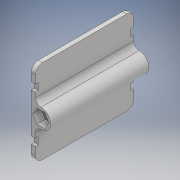
# Autodesk Inventor part: Soporte ESC
Saved by Autodesk Inventor 2019 (Build 230136000, 136)
## iProperties
Part Number: Soporte ESC
Material: Genérico
Document SubType Name: Modeling
Designer: beta3
Density: 1 g/cm^3
Appearance: Valor por defecto
Author: beta3
Autodesk Inventor part; units mm, degrees
ref_plane "YZ Plane" through (0, 0, 0) normal (1, 0, 0) x (0, 1, 0)
ref_plane "XZ Plane" through (0, 0, 0) normal (0, 1, 0) x (-1, 0, 0)
ref_plane "XY Plane" through (0, 0, 0) normal (0, 0, 1) x (1, 0, 0)
sketch "Boceto1" plane through (0, 0, 0) normal (0, 1, 0) x (-1, 0, 0)
  circle A0 centre (0, 0) radius 3.15
  line L0 (6.889, 30) -> (3.889, 30)
  line L1 (3.889, -30) -> (6.889, -30)
  line L2 (6.889, -30) -> (6.889, 30)
  line L3 (0, 0) -> (3.15, 0) construction
  arc A1 (0, 6.889) -> (0, -6.889) centre (0, 0) ccw
  line L4 (3.889, 30) -> (3.889, 10.7779)
  line L5 (3.889, -30) -> (3.889, -10.7779)
  arc A2 (0, 6.889) -> (3.889, 10.7779) centre (0, 10.7779) ccw
  arc A3 (3.889, -10.7779) -> (0, -6.889) centre (0, -10.7779) ccw
  line L6 (2.9445, 5.1) -> (5.889, 0) construction
  line L7 (5.889, 0) -> (2.9445, -5.1) construction
  line L8 (2.9445, -5.1) -> (-2.9445, -5.1) construction
  line L9 (-2.9445, -5.1) -> (-5.889, 0) construction
  line L10 (-5.889, 0) -> (-2.9445, 5.1) construction
  line L11 (-2.9445, 5.1) -> (2.9445, 5.1) construction
  line L12 (5.889, 0) -> (6.889, 0) construction
  line L13 (-5.889, 0) -> (-6.889, 0) construction
  line L14 (0, -10.7779) -> (0, 0) construction
  dimension "d0" = 6.3
  dimension "d3" = 10.2
  dimension "d4" = 1
  dimension "d5" = 3
  dimension "d12" = 60
  constraints: 30 end point, 7 point on circle, 4 symmetric about line, 4 tangent, 3 centre point, 3 coincident, 3 horizontal, 3 vertical, 1 collinear, 1 horizontal alignment, 1 midpoint, 1 parallel, 15 other
  measures "d3" distance between parallel lines of L8 L11
  measures "d4" distance of L6.end L12.end
  measures "d5" distance of L1.start L1.end
  measures "d12" distance of L1.end L0.start
extrude "Extrusión1" add sketch "Boceto1" along normal blind 70
sketch "Boceto2" plane through (0, 0, 0) normal (0, -1, 0) x (1, 0, 0)
  line L0 (-5.7735, 0) -> (-2.8868, 5)
  line L1 (-2.8868, 5) -> (2.8868, 5)
  line L2 (2.8868, 5) -> (5.7735, 0)
  line L3 (5.7735, 0) -> (2.8868, -5)
  line L4 (2.8868, -5) -> (-2.8868, -5)
  line L5 (-2.8868, -5) -> (-5.7735, 0)
  point P0 (0, 0)
  point P1 (0, 0)
  dimension "d8" = 10
  constraints: 12 end point, 1 coincident, 13 other
  measures "d8" distance between parallel lines of L4 L1
extrude "Extrusión2" cut sketch "Boceto2" against normal blind 6
sketch "Boceto4" plane through (-6.889, 0, -30) normal (-1, 0, 0) x (0, 0, 1)
  line L0 (10.7549, 2) -> (15.7549, 2)
  line L1 (15.7549, 2) -> (15.7549, 0)
  line L2 (15.7549, 0) -> (10.7549, 0)
  line L3 (10.7549, 0) -> (10.7549, 2)
  line L4 (44.2451, 2) -> (49.2451, 2)
  line L5 (49.2451, 2) -> (49.2451, 0)
  line L6 (49.2451, 0) -> (44.2451, 0)
  line L7 (44.2451, 0) -> (44.2451, 2)
  line L8 (0, 0) -> (60, 0) projected
  line L9 (30, 0) -> (30, 6) projected
  line L10 (30, 0) -> (30, 70) construction
  line L11 (0, 70) -> (60, 70) projected
  line L12 (30, 35) -> (1.5097, 35) construction
  line L13 (10.7549, 68) -> (15.7549, 68)
  line L14 (15.7549, 68) -> (15.7549, 70)
  line L15 (15.7549, 70) -> (10.7549, 70)
  line L16 (10.7549, 70) -> (10.7549, 68)
  line L17 (44.2451, 68) -> (49.2451, 68)
  line L18 (49.2451, 68) -> (49.2451, 70)
  line L19 (49.2451, 70) -> (44.2451, 70)
  line L20 (44.2451, 70) -> (44.2451, 68)
  point P0 (47.493, 22.347)
  dimension "d19" = 5
  dimension "d20" = 2
  constraints: 36 end point, 9 symmetric about line, 4 parallel, 3 horizontal, 2 equal length, 2 midpoint, 2 perpendicular, 1 point on line
  measures "d19" distance of L4.start L4.end
  measures "d20" distance of L6.end L4.start
extrude "Extrusión3" cut sketch "Boceto4" against normal up to next
fillet "Empalme1" radius 5 4 edges at (-5.389, 70, -30) (-5.389, 70, 30) (-5.389, 0, 30) (-5.389, 0, -30)
